Autodesk Fusion 360 part; units mm, degrees
note: some values were not read from the file. Set by a fixed rule: which sketch regions a step uses.
(part 2 of 2)
sketch "Sketch27" plane through (0, 0, 63.5) normal (0, 0, 1) x (1, 0, 0)
  circle A0 centre (20.7289, 22.871) radius 3.5
  circle A1 centre (-20.3538, 22.8395) radius 3.5
  line L0 (3.0966, 43.0743) -> (3.0966, 41.3657)
  line L1 (3.0966, 41.3657) -> (-3.0988, 41.3657)
  line L2 (-3.0988, 41.3657) -> (-3.0988, 43.0743)
  line L3 (-3.0988, 43.0743) -> (3.0966, 43.0743)
  line L4 (-2.5485, -40.6814) -> (-2.5485, -35.3439)
  line L5 (-2.5485, -35.3439) -> (2.5315, -35.3439)
  line L6 (2.5315, -35.3439) -> (2.5315, -40.6814)
  line L7 (2.5315, -40.6814) -> (-2.5485, -40.6814)
  arc A2 (-31.4879, -5.6993) -> (-31.3557, 6.9834) centre (-31.7467, 0.6454) ccw
  ellipse E0 centre (0, 0) end of major axis (0, 44.45) minor radius 31.75 (-31.4879, -5.6993) -> (31.4886, -5.6926) ccw
  arc A3 (31.355, 6.9901) -> (31.4886, -5.6926) centre (31.7466, 0.6522) ccw
  ellipse E1 centre (0, 0) end of major axis (0, 44.45) minor radius 31.75 (31.355, 6.9901) -> (-31.3557, 6.9834) ccw
  line L8 (7.6088, -16.0819) -> (16.3223, -16.0922)
  line L9 (16.3223, -16.0922) -> (16.3223, -33.833)
  line L10 (16.3223, -33.833) -> (2.3267, -33.8557)
  line L11 (2.3267, -33.8557) -> (-13.4085, -33.833)
  line L12 (-13.4085, -33.833) -> (-15.9357, -33.833)
  line L13 (-15.9357, -33.833) -> (-15.9357, -16.0922)
  line L14 (-15.9357, -16.0922) -> (-13.3958, -16.0922)
  line L15 (-13.3958, -16.0922) -> (-13.3957, -16.053)
  line L16 (-13.3957, -16.053) -> (-7.8668, -16.061)
  line L17 (-7.8668, -16.061) -> (-7.8564, -8.8494)
  line L18 (-7.8564, -8.8494) -> (-10.0299, -8.8463)
  line L19 (-10.0299, -8.8463) -> (-12.5699, -8.9534)
  line L20 (-12.5699, -8.9534) -> (-12.5699, -8.6333)
  line L21 (-12.5699, -8.6333) -> (-15.1099, -8.6009)
  line L22 (-15.1099, -8.6009) -> (-15.1099, 9.1877)
  arc A4 (-15.2005, 9.3115) -> (-15.1099, 9.1877) centre (-10.0299, 12.9977) ccw
  arc A5 (-15.1099, 16.9304) -> (-15.2005, 9.3115) centre (-15.1099, 13.1204) ccw
  line L23 (-15.1099, 16.9304) -> (-15.1099, 34.8417)
  line L24 (-15.1099, 34.8417) -> (-4.8867, 34.8417)
  line L25 (-4.8867, 34.8417) -> (-4.8867, 39.9217)
  line L26 (-4.8867, 39.9217) -> (5.2733, 39.9217)
  line L27 (5.2733, 39.9217) -> (5.2733, 34.8417)
  line L28 (5.2733, 34.8417) -> (15.4965, 34.8417)
  line L29 (15.4965, 34.8417) -> (15.4965, 16.7945)
  arc A6 (15.4965, 9.1715) -> (15.4965, 16.7945) centre (15.4965, 12.983) ccw
  line L30 (15.4965, 9.1715) -> (15.4965, -8.992)
  line L31 (15.4965, -8.992) -> (12.9565, -8.9595)
  line L32 (12.9565, -8.9595) -> (12.9565, -8.992)
  line L33 (12.9565, -8.992) -> (10.4165, -8.8757)
  line L34 (10.4165, -8.8757) -> (7.6191, -8.8717)
  line L35 (7.6191, -8.8717) -> (7.6088, -16.0819)
extrude "Extrude30" add sketch "Sketch27" against normal blind 2.794 contours L4 L5 L6 L7
sketch "Sketch28" plane through (0, 0, 63.5) normal (0, 0, 1) x (1, 0, 0)
  circle A0 centre (20.7289, 22.871) radius 3.5
  circle A1 centre (-20.3538, 22.8395) radius 3.5
  line L0 (3.0966, 43.0743) -> (3.0966, 41.3657)
  line L1 (3.0966, 41.3657) -> (-3.0988, 41.3657)
  line L2 (-3.0988, 41.3657) -> (-3.0988, 43.0743)
  line L3 (-3.0988, 43.0743) -> (3.0966, 43.0743)
  arc A2 (-31.4879, -5.6993) -> (-31.3557, 6.9834) centre (-31.7467, 0.6454) ccw
  ellipse E0 centre (0, 0) end of major axis (0, 44.45) minor radius 31.75 (-31.4879, -5.6993) -> (31.4886, -5.6926) ccw
  arc A3 (31.355, 6.9901) -> (31.4886, -5.6926) centre (31.7466, 0.6522) ccw
  ellipse E1 centre (0, 0) end of major axis (0, 44.45) minor radius 31.75 (31.355, 6.9901) -> (-31.3557, 6.9834) ccw
  line L4 (7.6088, -16.0819) -> (16.3223, -16.0922)
  line L5 (16.3223, -16.0922) -> (16.3223, -33.833)
  line L6 (16.3223, -33.833) -> (2.3267, -33.8557)
  line L7 (2.3267, -33.8557) -> (-13.4085, -33.833)
  line L8 (-13.4085, -33.833) -> (-15.9357, -33.833)
  line L9 (-15.9357, -33.833) -> (-15.9357, -16.0922)
  line L10 (-15.9357, -16.0922) -> (-13.3958, -16.0922)
  line L11 (-13.3958, -16.0922) -> (-13.3957, -16.053)
  line L12 (-13.3957, -16.053) -> (-7.8668, -16.061)
  line L13 (-7.8668, -16.061) -> (-7.8564, -8.8494)
  line L14 (-7.8564, -8.8494) -> (-10.0299, -8.8463)
  line L15 (-10.0299, -8.8463) -> (-12.5699, -8.9534)
  line L16 (-12.5699, -8.9534) -> (-12.5699, -8.6333)
  line L17 (-12.5699, -8.6333) -> (-15.1099, -8.6009)
  line L18 (-15.1099, -8.6009) -> (-15.1099, 9.1877)
  arc A4 (-15.2005, 9.3115) -> (-15.1099, 9.1877) centre (-10.0299, 12.9977) ccw
  arc A5 (-15.1099, 16.9304) -> (-15.2005, 9.3115) centre (-15.1099, 13.1204) ccw
  line L19 (-15.1099, 16.9304) -> (-15.1099, 34.8417)
  line L20 (-15.1099, 34.8417) -> (-4.8867, 34.8417)
  line L21 (-4.8867, 34.8417) -> (-4.8867, 39.9217)
  line L22 (-4.8867, 39.9217) -> (5.2733, 39.9217)
  line L23 (5.2733, 39.9217) -> (5.2733, 34.8417)
  line L24 (5.2733, 34.8417) -> (15.4965, 34.8417)
  line L25 (15.4965, 34.8417) -> (15.4965, 16.7945)
  arc A6 (15.4965, 9.1715) -> (15.4965, 16.7945) centre (15.4965, 12.983) ccw
  line L26 (15.4965, 9.1715) -> (15.4965, -8.992)
  line L27 (15.4965, -8.992) -> (12.9565, -8.9595)
  line L28 (12.9565, -8.9595) -> (12.9565, -8.992)
  line L29 (12.9565, -8.992) -> (10.4165, -8.8757)
  line L30 (10.4165, -8.8757) -> (7.6191, -8.8717)
  line L31 (7.6191, -8.8717) -> (7.6088, -16.0819)
  line L32 (0, 0) -> (0.0616, -38.0127)
  circle A7 centre (0.1123, -39.6352) radius 3.5
  dimension "d104" = 7
  measures "d104" diameter of A7
extrude "Extrude31" cut sketch "Sketch28" against normal blind 7 contours A7
sketch "Sketch29" plane through (0, 0, 63.5) normal (0, 0, 1) x (1, 0, 0)
  circle A0 centre (0.1123, -39.6352) radius 3.5
  circle A1 centre (20.7289, 22.871) radius 3.5
  circle A2 centre (-20.3538, 22.8395) radius 3.5
  line L0 (3.0966, 43.0743) -> (3.0966, 41.3657)
  line L1 (3.0966, 41.3657) -> (-3.0988, 41.3657)
  line L2 (-3.0988, 41.3657) -> (-3.0988, 43.0743)
  line L3 (-3.0988, 43.0743) -> (3.0966, 43.0743)
  arc A3 (-31.4879, -5.6993) -> (-31.3557, 6.9834) centre (-31.7467, 0.6454) ccw
  ellipse E0 centre (0, 0) end of major axis (0, 44.45) minor radius 31.75 (-31.4879, -5.6993) -> (31.4886, -5.6926) ccw
  arc A4 (31.355, 6.9901) -> (31.4886, -5.6926) centre (31.7466, 0.6522) ccw
  ellipse E1 centre (0, 0) end of major axis (0, 44.45) minor radius 31.75 (31.355, 6.9901) -> (-31.3557, 6.9834) ccw
  line L4 (7.6088, -16.0819) -> (16.3223, -16.0922)
  line L5 (16.3223, -16.0922) -> (16.3223, -33.833)
  line L6 (16.3223, -33.833) -> (2.3267, -33.8557)
  line L7 (2.3267, -33.8557) -> (-13.4085, -33.833)
  line L8 (-13.4085, -33.833) -> (-15.9357, -33.833)
  line L9 (-15.9357, -33.833) -> (-15.9357, -16.0922)
  line L10 (-15.9357, -16.0922) -> (-13.3958, -16.0922)
  line L11 (-13.3958, -16.0922) -> (-13.3957, -16.053)
  line L12 (-13.3957, -16.053) -> (-7.8668, -16.061)
  line L13 (-7.8668, -16.061) -> (-7.8564, -8.8494)
  line L14 (-7.8564, -8.8494) -> (-10.0299, -8.8463)
  line L15 (-10.0299, -8.8463) -> (-12.5699, -8.9534)
  line L16 (-12.5699, -8.9534) -> (-12.5699, -8.6333)
  line L17 (-12.5699, -8.6333) -> (-15.1099, -8.6009)
  line L18 (-15.1099, -8.6009) -> (-15.1099, 9.1877)
  arc A5 (-15.2005, 9.3115) -> (-15.1099, 9.1877) centre (-10.0299, 12.9977) ccw
  arc A6 (-15.1099, 16.9304) -> (-15.2005, 9.3115) centre (-15.1099, 13.1204) ccw
  line L19 (-15.1099, 16.9304) -> (-15.1099, 34.8417)
  line L20 (-15.1099, 34.8417) -> (-4.8867, 34.8417)
  line L21 (-4.8867, 34.8417) -> (-4.8867, 39.9217)
  line L22 (-4.8867, 39.9217) -> (5.2733, 39.9217)
  line L23 (5.2733, 39.9217) -> (5.2733, 34.8417)
  line L24 (5.2733, 34.8417) -> (15.4965, 34.8417)
  line L25 (15.4965, 34.8417) -> (15.4965, 16.7945)
  arc A7 (15.4965, 9.1715) -> (15.4965, 16.7945) centre (15.4965, 12.983) ccw
  line L26 (15.4965, 9.1715) -> (15.4965, -8.992)
  line L27 (15.4965, -8.992) -> (12.9565, -8.9595)
  line L28 (12.9565, -8.9595) -> (12.9565, -8.992)
  line L29 (12.9565, -8.992) -> (10.4165, -8.8757)
  line L30 (10.4165, -8.8757) -> (7.6191, -8.8717)
  line L31 (7.6191, -8.8717) -> (7.6088, -16.0819)
